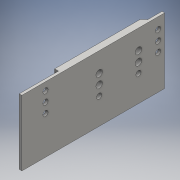
# Autodesk Inventor part: DrivenSideBallScrewSupport
Saved by Autodesk Inventor 2016 (Build 200138000, 138)
## iProperties
Created: 2017-10-24
Part Number: DrivenSideBallScrewSupport
Material: Generic
Document SubType Name: Modeling
Designer: m228540
Density: 1 g/cm^3
Appearance: Default
Author: m228540
Autodesk Inventor part; units mm, degrees
ref_plane "YZ Plane" through (0, 0, 0) normal (1, 0, 0) x (0, 1, 0)
ref_plane "XZ Plane" through (0, 0, 0) normal (0, 1, 0) x (-1, 0, 0)
ref_plane "XY Plane" through (0, 0, 0) normal (0, 0, 1) x (1, 0, 0)
sketch "Sketch1" plane through (0, 0, 0) normal (1, 0, 0) x (0, 1, 0)
  line L0 (109, 50) -> (-109, 50)
  line L1 (-109, 50) -> (-109, -50)
  line L2 (-109, -50) -> (109, -50)
  line L3 (109, -50) -> (109, 50)
  line L4 (109, 50) -> (-109, -50) construction
  line L5 (-109, 50) -> (109, -50) construction
  point P0 (0, 0)
  dimension "d0" = 100
  dimension "d1" = 218
  constraints: 12 end point, 2 midpoint, 2 parallel, 1 horizontal, 1 perpendicular
  measures "d0" distance of L0.end L1.end
  measures "d1" distance of L1.end L2.end
extrude "Extrusion1" add sketch "Sketch1" along normal mid plane 10
sketch "Sketch2" plane through (-5, -109, 50) normal (0, 0, 1) x (1, 0, 0)
  line L0 (0, 218) -> (10, 218) projected
  line L1 (6, 218) -> (6, 196)
  line L2 (6, 196) -> (0, 190)
  line L3 (0, 218) -> (0, 0) projected
  line L4 (6, 218) -> (0, 218)
  line L5 (0, 190) -> (0, 218)
  line L6 (0, 0) -> (10, 0) projected
  line L7 (6, 0) -> (6, 60)
  line L8 (6, 60) -> (0, 60)
  line L9 (6, 0) -> (0, 0)
  line L10 (0, 60) -> (0, 0)
  point P0 (5, 109)
  dimension "d5" = 4
  dimension "d6" = 22
  dimension "d7" = 135
  dimension "d8" = 60
  dimension "d10" = 4
  constraints: 16 end point, 4 collinear, 4 point on line, 2 vertical, 1 perpendicular
  measures "d5" distance of L0.end L1.start
  measures "d6" distance of L1.start L1.end
  measures "d7" angle of L1 L2
  measures "d8" distance of L7.start L7.end
  measures "d10" distance of L6.end L7.start
extrude "Extrusion2" cut sketch "Sketch2" against normal through all
sketch "Sketch3" plane through (5, 0, 0) normal (1, 0, 0) x (0, 0, -1)
  circle A0 centre (-38, -73) radius 4
  circle A1 centre (-23, -73) radius 4
  circle A2 centre (-8, -73) radius 4
  circle A3 centre (-33, 99) radius 4
  circle A4 centre (-18, 99) radius 4
  circle A5 centre (-3, 99) radius 4
  line L0 (-50, 109) -> (-50, -109) projected
  line L1 (-33, 99) -> (-18, 99) construction
  line L2 (-18, 99) -> (-3, 99) construction
  line L3 (50, 109) -> (-50, 109) projected
  line L4 (-38, -73) -> (-23, -73) construction
  line L5 (-23, -73) -> (-8, -73) construction
  line L6 (-50, -109) -> (50, -109) projected
  circle A6 centre (-20, 69) radius 5
  circle A7 centre (-5, 69) radius 5
  circle A8 centre (10, 69) radius 4
  circle A9 centre (-20, 9) radius 5
  circle A10 centre (-5, 9) radius 5
  circle A11 centre (10, 9) radius 4
  line L7 (-20, 69) -> (10, 69) construction
  line L8 (-20, 9) -> (10, 9) construction
  line L9 (-20, 9) -> (-20, 69) construction
  point P0 (0, 0)
  dimension "d13" = 8
  dimension "d14" = 8
  dimension "d15" = 17
  dimension "d16" = 15
  dimension "d17" = 15
  dimension "d18" = 10
  dimension "d19" = 12
  dimension "d20" = 15
  dimension "d21" = 15
  dimension "d22" = 36
  dimension "d23" = 10
  dimension "d24" = 8
  dimension "d25" = 40
  dimension "d26" = 30
  dimension "d27" = 15
  dimension "d28" = 15
  dimension "d29" = 60
  dimension "d30" = 15
  dimension "d31" = 15
  constraints: 14 end point, 12 centre point, 8 equal radius, 4 horizontal, 2 collinear, 2 midpoint, 1 vertical
  measures "d13" diameter of A3
  measures "d14" diameter of A5
  measures "d15" distance from line of L0 L1.start
  measures "d16" distance of L1.start L1.end
  measures "d17" distance of L2.end L1.end
  measures "d18" distance between parallel lines of L3 L1
  measures "d19" distance from line of L0 L4.start
  measures "d20" distance of L4.start L4.end
  measures "d21" distance of L4.end L5.end
  measures "d22" distance from line of L6 L4.start
  measures "d23" diameter of A6
  measures "d24" diameter of A8
  measures "d25" distance from line of L3 L7.start
  measures "d26" distance from line of L0 L7.start
  measures "d27" distance of L7.start A7.centre
  measures "d28" distance of L7.end A7.centre
  measures "d29" distance between parallel lines of L7 L8
  measures "d30" distance of A10.centre L8.start
  measures "d31" distance of L8.end A10.centre
extrude "Extrusion3" cut sketch "Sketch3" against normal through all
body "Solid1"
